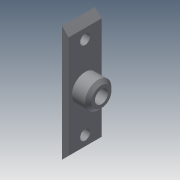
# Autodesk Inventor part: paka_packa
Saved by Autodesk Inventor 2015 (Build 190159000, 159)
## iProperties
Created: 2013-06-06
Part Number: paka_packa
Material: Generic
Document SubType Name: Modeling
Designer: idle-rug
Density: 1 g/cm^3
Appearance: Default
Author: idle-rug
Autodesk Inventor part; units mm, degrees
ref_plane "YZ Plane" through (0, 0, 0) normal (1, 0, 0) x (0, 1, 0)
ref_plane "XZ Plane" through (0, 0, 0) normal (0, 1, 0) x (-1, 0, 0)
ref_plane "XY Plane" through (0, 0, 0) normal (0, 0, 1) x (1, 0, 0)
sketch "Sketch1" plane through (0, 0, 0) normal (1, 0, 0) x (0, 1, 0)
  line L0 (5, -17.593) -> (-5, -17.593)
  line L1 (-5, -17.593) -> (-5, 17.593)
  line L2 (-5, 17.593) -> (5, 17.593)
  line L3 (5, 17.593) -> (5, -17.593)
  line L4 (5, -17.593) -> (-5, 17.593) construction
  line L5 (-5, -17.593) -> (5, 17.593) construction
  point P0 (0, 0)
  dimension "d0" = 35.186
  dimension "d2" = 10
  constraints: 12 end point, 2 midpoint, 2 parallel, 1 horizontal, 1 perpendicular
  measures "d0" distance of L0.end L1.end
  measures "d2" distance of L1.end L2.end
extrude "Extrusion1" add sketch "Sketch1" along normal blind 2
sketch "Sketch2" plane through (2, 0, 0) normal (1, 0, 0) x (0, 0, -1)
  circle A0 centre (0, 0) radius 4
  dimension "d5" = 8
  constraints: 1 centre point, 1 coincident
  measures "d5" diameter of A0
extrude "Extrusion2" add sketch "Sketch2" along normal blind 5
sketch "Sketch3" plane through (7, 0, 0) normal (1, 0, 0) x (0, 0, -1)
  circle A0 centre (0, 0) radius 4 projected
  circle A1 centre (0, 0) radius 2
  dimension "d8" = 4
  constraints: 1 centre point, 1 coincident
  measures "d8" diameter of A1
extrude "Extrusion3" cut sketch "Sketch3" against normal blind 7 contours A1
sketch "Sketch4" plane through (2, 0, 0) normal (1, 0, 0) x (0, 0, -1)
  line L0 (-17.593, 5) -> (-12.593, 5)
  line L1 (-12.593, 5) -> (-12.593, 0)
  line L2 (-12.593, 0) -> (-17.593, 0)
  line L3 (-17.593, 0) -> (-17.593, 5)
  line L4 (17.593, 5) -> (12.593, 5)
  line L5 (12.593, 5) -> (12.593, 0)
  line L6 (12.593, 0) -> (17.593, 0)
  line L7 (17.593, 0) -> (17.593, 5)
  circle A0 centre (-12.593, 0) radius 1.5
  circle A1 centre (12.593, 0) radius 1.5
  dimension "d11" = 5
  dimension "d12" = 5
  dimension "d13" = 3
  dimension "d14" = 3
  constraints: 16 end point, 4 parallel, 2 centre point, 2 coincident, 2 horizontal, 2 perpendicular
  measures "d11" distance of L1.end L2.end
  measures "d12" distance of L6.end L5.end
  measures "d13" diameter of A0
  measures "d14" diameter of A1
extrude "Extrusion4" cut sketch "Sketch4" against normal blind 2 contours A0 L2 L1 | L1 L2 A0 | A1 L6 L5 | L5 L6 A1
chamfer "Chamfer1" distance 1 angle 45 1 edges at (7, 0, 4)
chamfer "Chamfer2" distance 2 angle 45 2 edges at (2, 0, -17.593) (2, 0, 17.593)
body "Solid1"
